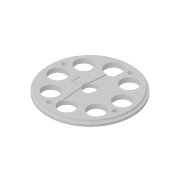
# Autodesk Inventor part: Left_Wheel_Disk
Saved by Autodesk Inventor 2019 (Build 230136000, 136)
## iProperties
Created: 2021-06-26
Part Number: Left_Wheel_Disk
Material: Generic
Document SubType Name: Modeling
Designer: Oudenas
Density: 1 g/cm^3
Appearance: Default
Author: Oudenas
Autodesk Inventor part; units mm, degrees
ref_plane "YZ Plane" through (0, 0, 0) normal (1, 0, 0) x (0, 1, 0)
ref_plane "XZ Plane" through (0, 0, 0) normal (0, 1, 0) x (-1, 0, 0)
ref_plane "XY Plane" through (0, 0, 0) normal (0, 0, 1) x (1, 0, 0)
sketch "Sketch1" plane through (0, 0, 0) normal (0, 1, 0) x (-1, 0, 0)
  circle A0 centre (0, 0) radius 28
  dimension "d0" = 56
  constraints: 1 centre point, 1 coincident
  measures "d0" diameter of A0
extrude "Extrusion1" add sketch "Sketch1" along normal blind 3
sketch "Sketch2" plane through (0, 3, 0) normal (0, 1, 0) x (1, 0, 0)
  circle A0 centre (0, 0) radius 3.5
  dimension "d51" = 7
  constraints: 1 centre point
  measures "d51" diameter of A0
extrude "Extrusion2" cut sketch "Sketch2" against normal blind 3
sketch "Sketch5" plane through (0, 3, 0) normal (0, 1, 0) x (1, 0, 0)
  circle A0 centre (0, 0) radius 22.5 construction
  circle A1 centre (5.0614, 21.9233) radius 1.5
  circle A2 centre (21.9233, -5.0614) radius 1.5
  circle A3 centre (-5.0614, -21.9233) radius 1.5
  circle A4 centre (-21.9233, 5.0614) radius 1.5
  line L0 (0, 0) -> (-21.9233, 5.0614)
  line L1 (0, 0) -> (5.0614, 21.9233)
  line L2 (0, 0) -> (21.9233, -5.0614)
  line L3 (0, 0) -> (-5.0614, -21.9233)
  circle A5 centre (0, 0) radius 28 projected
  line L4 (-28, 0) -> (28, 0) construction
  line L5 (0, -28) -> (0, 28) construction
  dimension "d27" = 45
  dimension "d28" = 3
  dimension "d29" = 3
  dimension "d30" = 3
  dimension "d31" = 3
  dimension "d57" = 13
  dimension "d58" = 13
  constraints: 12 end point, 8 point on circle, 5 centre point, 2 point on line, 1 coincident, 1 perpendicular
  measures "d27" diameter of A0
  measures "d28" diameter of A1
  measures "d29" diameter of A2
  measures "d30" diameter of A3
  measures "d31" diameter of A4
  measures "d57" angle of L1 L5
  measures "d58" angle of L4 L2
extrude "Extrusion5" cut sketch "Sketch5" against normal blind 3 contours A1 | A2 | A3 | A4
fillet "Fillet1" radius 1.5 1 edges at (28, 3, 0) inverted yes
sketch "Sketch6" plane through (0, 3, 0) normal (0, 1, 0) x (1, 0, 0)
  circle A0 centre (0, 0) radius 26.5 construction
  circle A1 centre (0, 0) radius 4.5 construction
  circle A2 centre (0, 0) radius 6.25 construction
  circle A3 centre (-21.9233, 5.0614) radius 1.5 construction
  circle A4 centre (0, 0) radius 22.5 construction
  circle A5 centre (0, 0) radius 18.75 construction
  line L0 (0, 0) -> (-18.509, -2.9965) construction
  circle A6 centre (-18.509, -2.9965) radius 5.25
  dimension "d37" = 37.5
  dimension "d62" = 8.5
  dimension "d63" = 10.5
  constraints: 6 coincident, 4 centre point, 2 end point, 6 other
  measures "d62" distance from line of L0 A3.centre
  measures "d63" diameter of A6
extrude "Extrusion7" cut sketch "Sketch6" against normal blind 3
pattern_circular "Circular Pattern2" count 8 over 360 about axis through (0, 3, 0) along (0, 1, 0) of "Extrusion7"
sketch "Sketch7" plane through (0, 3, 0) normal (0, 1, 0) x (1, 0, 0)
  circle A0 centre (0, 0) radius 3.5 construction
  line L0 (0, -15) -> (0, 15) construction
  arc A1 (-2, -15) -> (2, -15) centre (0, -15) ccw
  arc A2 (2, 15) -> (-2, 15) centre (0, 15) ccw
  line L1 (2, 15) -> (3.4822, 0.3524)
  circle A3 centre (0, 0) radius 3.5 projected
  line L2 (2, -15) -> (3.4822, -0.3524)
  line L3 (-2, -15) -> (-3.4822, -0.3524)
  line L4 (-2, 15) -> (-3.4822, 0.3524)
  dimension "d52" = 7
  dimension "d53" = 15
  dimension "d54" = 4
  constraints: 12 end point, 8 point on circle, 4 tangent, 3 centre point, 1 coincident, 1 midpoint, 1 vertical
  measures "d52" diameter of A0
  measures "d53" distance of A0.centre L0.end
  measures "d54" diameter of A2
extrude "Extrusion8" cut sketch "Sketch7" against normal blind 0.7 contours L3 A3 L2 A1 | L4 A2 L1 A3
sketch "Sketch8" plane through (0, 0, 0) normal (0, -1, 0) x (1, 0, 0)
  circle A0 centre (0, 0) radius 4
  dimension "d64" = 8
  constraints: 1 centre point, 1 coincident
  measures "d64" diameter of A0
extrude "Extrusion9" cut sketch "Sketch8" against normal blind 3
sketch "Sketch9" plane through (0, 3, 0) normal (0, 1, 0) x (1, 0, 0)
  line L0 (-10.6108, 3.0214) -> (-5.7422, 3.0214) construction
  line L1 (-5.7422, 3.0214) -> (-5.7422, -3.0786) construction
  line L2 (-5.7422, -3.0786) -> (-10.6108, -3.0786) construction
  line L3 (-10.6108, -3.0786) -> (-10.6108, 3.0214) construction
  spline S0 degree 2 poles (-5.8167, -2.5631) (-5.8167, -2.7005) (-5.8453, -2.8953) (-5.9026, -3.0213) (-5.9885, -3.0786) (-6.0458, -3.0786) knots 0 0 0 1 2 3 4 4 4
  line L4 (-6.0458, -3.0786) -> (-9.3793, -3.0786)
  spline S1 degree 2 poles (-9.3793, -3.0786) (-9.5626, -3.0786) (-9.8203, -2.8953) (-9.8203, -2.6891) knots 0 0 0 1 2 2 2
  line L5 (-9.8203, -2.6891) -> (-9.8203, 2.8267)
  spline S2 degree 2 poles (-9.8203, 2.8267) (-9.8203, 2.8725) (-9.7459, 2.947) (-9.574, 2.9928) (-9.2877, 3.0214) (-9.0757, 3.0214) knots 0 0 0 1 2 3 4 4 4
  spline S3 degree 2 poles (-9.0757, 3.0214) (-8.8581, 3.0214) (-8.5774, 2.9928) (-8.4056, 2.947) (-8.3311, 2.8725) (-8.3311, 2.8267) knots 0 0 0 1 2 3 4 4 4
  line L6 (-8.3311, 2.8267) -> (-8.3311, -2.059)
  line L7 (-8.3311, -2.059) -> (-6.0458, -2.059)
  spline S4 degree 2 poles (-6.0458, -2.059) (-5.9885, -2.059) (-5.9026, -2.1106) (-5.8453, -2.2309) (-5.8167, -2.4199) (-5.8167, -2.5631) knots 0 0 0 1 2 3 4 4 4
  point P0 (0, 0)
  constraints: 2 other
extrude "Extrusion10" cut sketch "Sketch9" against normal blind 0.5
fillet "Fillet2" radius 0.4 1 edges at (-8.3311, 2.75, 2.059)
body "Solid1"
